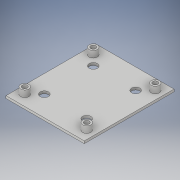
# Autodesk Inventor part: Box2_Buttom
Saved by Autodesk Inventor 2017 (Build 210142000, 142)
## iProperties
Created: 2017-11-17
Part Number: Box2_Buttom
Material: Generic
Document SubType Name: Modeling
Designer: Arthur Bondar
Density: 1 g/cm^3
Appearance: Default
Author: Arthur Bondar
Autodesk Inventor part; units mm, degrees
ref_plane "YZ Plane" through (0, 0, 0) normal (1, 0, 0) x (0, 1, 0)
ref_plane "XZ Plane" through (0, 0, 0) normal (0, 1, 0) x (-1, 0, 0)
ref_plane "XY Plane" through (0, 0, 0) normal (0, 0, 1) x (1, 0, 0)
sketch "Sketch1" plane through (0, 0, 0) normal (0, 1, 0) x (-1, 0, 0)
  line L0 (-24, 27.5) -> (24, 27.5)
  line L1 (24, 27.5) -> (24, -27.5)
  line L2 (24, -27.5) -> (-24, -27.5)
  line L3 (-24, -27.5) -> (-24, 27.5)
  dimension "d13" = 48
  dimension "d14" = 55
  constraints: 8 end point, 2 parallel, 1 horizontal, 1 perpendicular
  measures "d13" distance of L1.end L2.end
  measures "d14" distance of L0.end L1.end
extrude "Extrusion1" add sketch "Sketch1" along normal blind 1.5
sketch "Sketch2" plane through (0, 1.5, 0) normal (0, 1, 0) x (1, 0, 0)
  circle A0 centre (19, 21) radius 2.5
  circle A1 centre (19, -21) radius 2.5
  circle A2 centre (-19, -21) radius 2.5
  circle A3 centre (-19, 21) radius 2.5
  circle A4 centre (-13, -15) radius 2.5
  circle A5 centre (13, -15) radius 2.5
  circle A6 centre (13, 15) radius 2.5
  circle A7 centre (-13, 15) radius 2.5
  circle A8 centre (19, -21) radius 1.5
  circle A9 centre (19, 21) radius 1.5
  circle A10 centre (-19, 21) radius 1.5
  circle A11 centre (-19, -21) radius 1.5
  dimension "d47" = 3
  dimension "d48" = 3
  dimension "d50" = 3
  constraints: 12 centre point, 4 coincident
  measures "d47" diameter of A8
  measures "d48" diameter of A9
  measures "d50" diameter of A11
extrude "Extrusion2" add sketch "Sketch2" along normal blind 4 contours A0 | A1 | A2 | A3
sketch "Sketch3" plane through (0, 1.5, 0) normal (0, 1, 0) x (1, 0, 0)
  circle A0 centre (-13, -15) radius 2.5
  circle A1 centre (13, -15) radius 2.5
  circle A2 centre (13, 15) radius 2.5
  circle A3 centre (-13, 15) radius 2.5
  point P0 (0, 0)
  constraints: 4 centre point
extrude "Extrusion3" cut sketch "Sketch3" against normal through all
body "Solid1"
